Autodesk Fusion 360 part; units mm, degrees
note: some values were not read from the file. Set by a fixed rule: which sketch regions a step uses.
(part 2 of 2)
sketch "Sketch14" plane through (0, 1.4, 0) normal (0, 1, 0) x (-1, 0, 0)
  circle A0 centre (-36, -115) radius 1.625
  circle A1 centre (-3.5, -133) radius 1.625
  line L0 (0, -38.25) -> (-124, -38.25)
  line L1 (-124, -38.25) -> (-124, -58)
  line L2 (-124, -58) -> (-102, -112)
  line L3 (-102, -112) -> (-96.5, -117.5)
  line L4 (-96.5, -117.5) -> (-25, -136.5)
  line L5 (-25, -136.5) -> (-2.5, -136.5)
  line L6 (-2.5, -136.5) -> (0, -134)
  line L7 (0, -134) -> (0, -38.25)
  line L8 (-68.85, -56.1) -> (-82.85, -56.1)
  line L9 (-82.85, -56.1) -> (-82.85, -42.1)
  line L10 (-82.85, -42.1) -> (-68.85, -42.1)
  line L11 (-68.85, -42.1) -> (-68.85, -56.1)
  line L12 (-51, -56.1) -> (-65, -56.1)
  line L13 (-65, -56.1) -> (-65, -42.1)
  line L14 (-65, -42.1) -> (-51, -42.1)
  line L15 (-51, -42.1) -> (-51, -56.1)
  line L16 (-86.7, -56.1) -> (-100.7, -56.1)
  line L17 (-100.7, -56.1) -> (-100.7, -42.1)
  line L18 (-100.7, -42.1) -> (-86.7, -42.1)
  line L19 (-86.7, -42.1) -> (-86.7, -56.1)
  line L20 (-21.075, -56.1) -> (-35.075, -56.1)
  line L21 (-35.075, -56.1) -> (-35.075, -42.1)
  line L22 (-35.075, -42.1) -> (-21.075, -42.1)
  line L23 (-21.075, -42.1) -> (-21.075, -56.1)
  line L24 (-104.55, -56.1) -> (-118.55, -56.1)
  line L25 (-118.55, -56.1) -> (-118.55, -42.1)
  line L26 (-118.55, -42.1) -> (-104.55, -42.1)
  line L27 (-104.55, -42.1) -> (-104.55, -56.1)
  line L28 (-62.7, -73.95) -> (-76.7, -73.95)
  line L29 (-76.7, -73.95) -> (-76.7, -59.95)
  line L30 (-76.7, -59.95) -> (-62.7, -59.95)
  line L31 (-62.7, -59.95) -> (-62.7, -73.95)
  line L32 (-44.85, -59.95) -> (-44.85, -73.95)
  line L33 (-44.85, -73.95) -> (-58.85, -73.95)
  line L34 (-58.85, -73.95) -> (-58.85, -59.95)
  line L35 (-58.85, -59.95) -> (-44.85, -59.95)
  line L36 (-80.55, -73.95) -> (-94.55, -73.95)
  line L37 (-94.55, -73.95) -> (-94.55, -59.95)
  line L38 (-94.55, -59.95) -> (-80.55, -59.95)
  line L39 (-80.55, -59.95) -> (-80.55, -73.95)
  line L40 (-19.675, -73.95) -> (-33.675, -73.95)
  line L41 (-33.675, -73.95) -> (-33.675, -59.95)
  line L42 (-33.675, -59.95) -> (-19.675, -59.95)
  line L43 (-19.675, -59.95) -> (-19.675, -73.95)
  line L44 (-98.4, -59.95) -> (-98.4, -73.95)
  line L45 (-98.4, -73.95) -> (-112.4, -73.95)
  line L46 (-112.4, -73.95) -> (-112.4, -59.95)
  line L47 (-112.4, -59.95) -> (-98.4, -59.95)
  line L48 (-68.6, -91.85) -> (-68.6, -77.85)
  line L49 (-68.6, -77.85) -> (-54.6, -77.85)
  line L50 (-54.6, -77.85) -> (-54.6, -91.85)
  line L51 (-54.6, -91.85) -> (-68.6, -91.85)
  line L52 (-50.75, -91.85) -> (-50.75, -77.85)
  line L53 (-50.75, -77.85) -> (-36.75, -77.85)
  line L54 (-36.75, -77.85) -> (-36.75, -91.85)
  line L55 (-36.75, -91.85) -> (-50.75, -91.85)
  line L56 (-86.45, -91.85) -> (-86.45, -77.85)
  line L57 (-86.45, -77.85) -> (-72.45, -77.85)
  line L58 (-72.45, -77.85) -> (-72.45, -91.85)
  line L59 (-72.45, -91.85) -> (-86.45, -91.85)
  line L60 (-28.325, -77.85) -> (-14.325, -77.85)
  line L61 (-14.325, -77.85) -> (-14.325, -91.85)
  line L62 (-14.325, -91.85) -> (-28.325, -91.85)
  line L63 (-28.325, -91.85) -> (-28.325, -77.85)
  line L64 (-104.3, -91.85) -> (-104.3, -77.85)
  line L65 (-104.3, -77.85) -> (-90.3, -77.85)
  line L66 (-90.3, -77.85) -> (-90.3, -91.85)
  line L67 (-90.3, -91.85) -> (-104.3, -91.85)
  line L68 (-44.7, -95.65) -> (-44.7, -109.65)
  line L69 (-44.7, -109.65) -> (-58.7, -109.65)
  line L70 (-58.7, -109.65) -> (-58.7, -95.65)
  line L71 (-58.7, -95.65) -> (-44.7, -95.65)
  line L72 (-26.85, -95.65) -> (-26.85, -109.65)
  line L73 (-26.85, -109.65) -> (-40.85, -109.65)
  line L74 (-40.85, -109.65) -> (-40.85, -95.65)
  line L75 (-40.85, -95.65) -> (-26.85, -95.65)
  line L76 (-62.55, -95.65) -> (-62.55, -109.65)
  line L77 (-62.55, -109.65) -> (-76.55, -109.65)
  line L78 (-76.55, -109.65) -> (-76.55, -95.65)
  line L79 (-76.55, -95.65) -> (-62.55, -95.65)
  line L80 (-9, -95.65) -> (-9, -109.65)
  line L81 (-9, -109.65) -> (-23, -109.65)
  line L82 (-23, -109.65) -> (-23, -95.65)
  line L83 (-23, -95.65) -> (-9, -95.65)
  line L84 (-80.4, -95.65) -> (-80.4, -109.65)
  line L85 (-80.4, -109.65) -> (-94.4, -109.65)
  line L86 (-94.4, -109.65) -> (-94.4, -95.65)
  line L87 (-94.4, -95.65) -> (-80.4, -95.65)
  line L88 (-9, -113.5) -> (-9, -127.5)
  line L89 (-9, -127.5) -> (-23, -127.5)
  line L90 (-23, -127.5) -> (-23, -113.5)
  line L91 (-23, -113.5) -> (-9, -113.5)
  line L92 (0, -134) -> (0, -136.5)
  line L93 (0, -136.5) -> (-100, -136.5)
  line L94 (-100, -136.5) -> (-100, -97.5)
  line L95 (0, -136.5) -> (-110.5, -136.5)
  line L96 (-110.5, -136.5) -> (-110.5, -79.5)
  line L97 (0, -136.5) -> (-115, -136.5)
  line L98 (-115, -136.5) -> (-115, -62)
  circle A2 centre (-100, -97.5) radius 1.625
  circle A3 centre (-110.5, -79.5) radius 1.625
  circle A4 centre (-115, -62) radius 1.625
  line L99 (0, -67) -> (-23.5, -67)
  dimension "d114" = 100
  dimension "d115" = 39
  dimension "d116" = 110.5
  dimension "d117" = 57
  dimension "d118" = 74.5
  dimension "d119" = 3.25
  dimension "d120" = 3.25
  dimension "d121" = 3.25
  dimension "d122" = 23.5
  constraint coincident L6.end L7.start
  constraint perpendicular L5 L92
  constraint perpendicular L92 L93
  constraint perpendicular L93 L94
  constraint perpendicular L94 L95
  constraint perpendicular L95 L96
  constraint perpendicular L92 L97
  constraint perpendicular L97 L98
  constraint coincident L94.end A2.centre
  constraint coincident L96.end A3.centre
  constraint coincident L98.end A4.centre
  constraint coincident L7 L99.start
  constraint perpendicular L7 L99
  measures "d114" distance of L92.end L93.end
  measures "d115" distance of L93.end L94.end
  measures "d116" distance of L92.end L95.end
  measures "d117" distance of L95.end L96.end
  measures "d118" distance of L97.end L98.end
  measures "d119" diameter of A2
  measures "d120" diameter of A3
  measures "d121" diameter of A4
  measures "d122" distance of L99.start L99.end
extrude "Extrude14" cut sketch "Sketch14" against normal blind 5 contours A2 | A3 | A4
sketch "Sketch15" plane through (0, 1.4, 0) normal (0, 1, 0) x (-1, 0, 0)
  circle A0 centre (-100, -97.5) radius 1.625
  circle A1 centre (-110.5, -79.5) radius 1.625
  circle A2 centre (-115, -62) radius 1.625
  circle A3 centre (-36, -115) radius 1.625
  circle A4 centre (-3.5, -133) radius 1.625
  line L0 (0, -38.25) -> (-124, -38.25)
  line L1 (-124, -38.25) -> (-124, -58)
  line L2 (-124, -58) -> (-102, -112)
  line L3 (-102, -112) -> (-96.5, -117.5)
  line L4 (-96.5, -117.5) -> (-25, -136.5)
  line L5 (-25, -136.5) -> (-2.5, -136.5)
  line L6 (-2.5, -136.5) -> (0, -134)
  line L7 (0, -134) -> (0, -38.25)
  line L8 (-68.85, -56.1) -> (-82.85, -56.1)
  line L9 (-82.85, -56.1) -> (-82.85, -42.1)
  line L10 (-82.85, -42.1) -> (-68.85, -42.1)
  line L11 (-68.85, -42.1) -> (-68.85, -56.1)
  line L12 (-51, -56.1) -> (-65, -56.1)
  line L13 (-65, -56.1) -> (-65, -42.1)
  line L14 (-65, -42.1) -> (-51, -42.1)
  line L15 (-51, -42.1) -> (-51, -56.1)
  line L16 (-86.7, -56.1) -> (-100.7, -56.1)
  line L17 (-100.7, -56.1) -> (-100.7, -42.1)
  line L18 (-100.7, -42.1) -> (-86.7, -42.1)
  line L19 (-86.7, -42.1) -> (-86.7, -56.1)
  line L20 (-21.075, -56.1) -> (-35.075, -56.1)
  line L21 (-35.075, -56.1) -> (-35.075, -42.1)
  line L22 (-35.075, -42.1) -> (-21.075, -42.1)
  line L23 (-21.075, -42.1) -> (-21.075, -56.1)
  line L24 (-104.55, -56.1) -> (-118.55, -56.1)
  line L25 (-118.55, -56.1) -> (-118.55, -42.1)
  line L26 (-118.55, -42.1) -> (-104.55, -42.1)
  line L27 (-104.55, -42.1) -> (-104.55, -56.1)
  line L28 (-62.7, -73.95) -> (-76.7, -73.95)
  line L29 (-76.7, -73.95) -> (-76.7, -59.95)
  line L30 (-76.7, -59.95) -> (-62.7, -59.95)
  line L31 (-62.7, -59.95) -> (-62.7, -73.95)
  line L32 (-44.85, -59.95) -> (-44.85, -73.95)
  line L33 (-44.85, -73.95) -> (-58.85, -73.95)
  line L34 (-58.85, -73.95) -> (-58.85, -59.95)
  line L35 (-58.85, -59.95) -> (-44.85, -59.95)
  line L36 (-80.55, -73.95) -> (-94.55, -73.95)
  line L37 (-94.55, -73.95) -> (-94.55, -59.95)
  line L38 (-94.55, -59.95) -> (-80.55, -59.95)
  line L39 (-80.55, -59.95) -> (-80.55, -73.95)
  line L40 (-19.675, -73.95) -> (-33.675, -73.95)
  line L41 (-33.675, -73.95) -> (-33.675, -59.95)
  line L42 (-33.675, -59.95) -> (-19.675, -59.95)
  line L43 (-19.675, -59.95) -> (-19.675, -73.95)
  line L44 (-98.4, -59.95) -> (-98.4, -73.95)
  line L45 (-98.4, -73.95) -> (-112.4, -73.95)
  line L46 (-112.4, -73.95) -> (-112.4, -59.95)
  line L47 (-112.4, -59.95) -> (-98.4, -59.95)
  line L48 (-68.6, -91.85) -> (-68.6, -77.85)
  line L49 (-68.6, -77.85) -> (-54.6, -77.85)
  line L50 (-54.6, -77.85) -> (-54.6, -91.85)
  line L51 (-54.6, -91.85) -> (-68.6, -91.85)
  line L52 (-50.75, -91.85) -> (-50.75, -77.85)
  line L53 (-50.75, -77.85) -> (-36.75, -77.85)
  line L54 (-36.75, -77.85) -> (-36.75, -91.85)
  line L55 (-36.75, -91.85) -> (-50.75, -91.85)
  line L56 (-86.45, -91.85) -> (-86.45, -77.85)
  line L57 (-86.45, -77.85) -> (-72.45, -77.85)
  line L58 (-72.45, -77.85) -> (-72.45, -91.85)
  line L59 (-72.45, -91.85) -> (-86.45, -91.85)
  line L60 (-28.325, -77.85) -> (-14.325, -77.85)
  line L61 (-14.325, -77.85) -> (-14.325, -91.85)
  line L62 (-14.325, -91.85) -> (-28.325, -91.85)
  line L63 (-28.325, -91.85) -> (-28.325, -77.85)
  line L64 (-104.3, -91.85) -> (-104.3, -77.85)
  line L65 (-104.3, -77.85) -> (-90.3, -77.85)
  line L66 (-90.3, -77.85) -> (-90.3, -91.85)
  line L67 (-90.3, -91.85) -> (-104.3, -91.85)
  line L68 (-44.7, -95.65) -> (-44.7, -109.65)
  line L69 (-44.7, -109.65) -> (-58.7, -109.65)
  line L70 (-58.7, -109.65) -> (-58.7, -95.65)
  line L71 (-58.7, -95.65) -> (-44.7, -95.65)
  line L72 (-26.85, -95.65) -> (-26.85, -109.65)
  line L73 (-26.85, -109.65) -> (-40.85, -109.65)
  line L74 (-40.85, -109.65) -> (-40.85, -95.65)
  line L75 (-40.85, -95.65) -> (-26.85, -95.65)
  line L76 (-62.55, -95.65) -> (-62.55, -109.65)
  line L77 (-62.55, -109.65) -> (-76.55, -109.65)
  line L78 (-76.55, -109.65) -> (-76.55, -95.65)
  line L79 (-76.55, -95.65) -> (-62.55, -95.65)
  line L80 (-9, -95.65) -> (-9, -109.65)
  line L81 (-9, -109.65) -> (-23, -109.65)
  line L82 (-23, -109.65) -> (-23, -95.65)
  line L83 (-23, -95.65) -> (-9, -95.65)
  line L84 (-80.4, -95.65) -> (-80.4, -109.65)
  line L85 (-80.4, -109.65) -> (-94.4, -109.65)
  line L86 (-94.4, -109.65) -> (-94.4, -95.65)
  line L87 (-94.4, -95.65) -> (-80.4, -95.65)
  line L88 (-9, -113.5) -> (-9, -127.5)
  line L89 (-9, -127.5) -> (-23, -127.5)
  line L90 (-23, -127.5) -> (-23, -113.5)
  line L91 (-23, -113.5) -> (-9, -113.5)
extrude "Extrude15" add sketch "Sketch15" against normal blind 1.4 contours L28 L29 L30 L31 | L32 L33 L34 L35 | L36 L37 L38 L39 | L40 L41 L42 L43 | L44 L45 L46 L47
sketch "Sketch16" plane through (0, 1.4, 0) normal (0, 1, 0) x (-1, 0, 0)
  circle A0 centre (-100, -97.5) radius 1.625
  circle A1 centre (-110.5, -79.5) radius 1.625
  circle A2 centre (-115, -62) radius 1.625
  circle A3 centre (-36, -115) radius 1.625
  circle A4 centre (-3.5, -133) radius 1.625
  line L0 (0, -38.25) -> (-124, -38.25)
  line L1 (-124, -38.25) -> (-124, -58)
  line L2 (-124, -58) -> (-102, -112)
  line L3 (-102, -112) -> (-96.5, -117.5)
  line L4 (-96.5, -117.5) -> (-25, -136.5)
  line L5 (-25, -136.5) -> (-2.5, -136.5)
  line L6 (-2.5, -136.5) -> (0, -134)
  line L7 (0, -134) -> (0, -38.25)
  line L8 (-68.85, -56.1) -> (-82.85, -56.1)
  line L9 (-82.85, -56.1) -> (-82.85, -42.1)
  line L10 (-82.85, -42.1) -> (-68.85, -42.1)
  line L11 (-68.85, -42.1) -> (-68.85, -56.1)
  line L12 (-51, -56.1) -> (-65, -56.1)
  line L13 (-65, -56.1) -> (-65, -42.1)
  line L14 (-65, -42.1) -> (-51, -42.1)
  line L15 (-51, -42.1) -> (-51, -56.1)
  line L16 (-86.7, -56.1) -> (-100.7, -56.1)
  line L17 (-100.7, -56.1) -> (-100.7, -42.1)
  line L18 (-100.7, -42.1) -> (-86.7, -42.1)
  line L19 (-86.7, -42.1) -> (-86.7, -56.1)
  line L20 (-21.075, -56.1) -> (-35.075, -56.1)
  line L21 (-35.075, -56.1) -> (-35.075, -42.1)
  line L22 (-35.075, -42.1) -> (-21.075, -42.1)
  line L23 (-21.075, -42.1) -> (-21.075, -56.1)
  line L24 (-104.55, -56.1) -> (-118.55, -56.1)
  line L25 (-118.55, -56.1) -> (-118.55, -42.1)
  line L26 (-118.55, -42.1) -> (-104.55, -42.1)
  line L27 (-104.55, -42.1) -> (-104.55, -56.1)
  line L28 (-68.6, -91.85) -> (-68.6, -77.85)
  line L29 (-68.6, -77.85) -> (-54.6, -77.85)
  line L30 (-54.6, -77.85) -> (-54.6, -91.85)
  line L31 (-54.6, -91.85) -> (-68.6, -91.85)
  line L32 (-50.75, -91.85) -> (-50.75, -77.85)
  line L33 (-50.75, -77.85) -> (-36.75, -77.85)
  line L34 (-36.75, -77.85) -> (-36.75, -91.85)
  line L35 (-36.75, -91.85) -> (-50.75, -91.85)
  line L36 (-86.45, -91.85) -> (-86.45, -77.85)
  line L37 (-86.45, -77.85) -> (-72.45, -77.85)
  line L38 (-72.45, -77.85) -> (-72.45, -91.85)
  line L39 (-72.45, -91.85) -> (-86.45, -91.85)
  line L40 (-28.325, -77.85) -> (-14.325, -77.85)
  line L41 (-14.325, -77.85) -> (-14.325, -91.85)
  line L42 (-14.325, -91.85) -> (-28.325, -91.85)
  line L43 (-28.325, -91.85) -> (-28.325, -77.85)
  line L44 (-104.3, -91.85) -> (-104.3, -77.85)
  line L45 (-104.3, -77.85) -> (-90.3, -77.85)
  line L46 (-90.3, -77.85) -> (-90.3, -91.85)
  line L47 (-90.3, -91.85) -> (-104.3, -91.85)
  line L48 (-44.7, -95.65) -> (-44.7, -109.65)
  line L49 (-44.7, -109.65) -> (-58.7, -109.65)
  line L50 (-58.7, -109.65) -> (-58.7, -95.65)
  line L51 (-58.7, -95.65) -> (-44.7, -95.65)
  line L52 (-26.85, -95.65) -> (-26.85, -109.65)
  line L53 (-26.85, -109.65) -> (-40.85, -109.65)
  line L54 (-40.85, -109.65) -> (-40.85, -95.65)
  line L55 (-40.85, -95.65) -> (-26.85, -95.65)
  line L56 (-62.55, -95.65) -> (-62.55, -109.65)
  line L57 (-62.55, -109.65) -> (-76.55, -109.65)
  line L58 (-76.55, -109.65) -> (-76.55, -95.65)
  line L59 (-76.55, -95.65) -> (-62.55, -95.65)
  line L60 (-9, -95.65) -> (-9, -109.65)
  line L61 (-9, -109.65) -> (-23, -109.65)
  line L62 (-23, -109.65) -> (-23, -95.65)
  line L63 (-23, -95.65) -> (-9, -95.65)
  line L64 (-80.4, -95.65) -> (-80.4, -109.65)
  line L65 (-80.4, -109.65) -> (-94.4, -109.65)
  line L66 (-94.4, -109.65) -> (-94.4, -95.65)
  line L67 (-94.4, -95.65) -> (-80.4, -95.65)
  line L68 (-9, -113.5) -> (-9, -127.5)
  line L69 (-9, -127.5) -> (-23, -127.5)
  line L70 (-23, -127.5) -> (-23, -113.5)
  line L71 (-23, -113.5) -> (-9, -113.5)
  line L72 (0, -66.975) -> (-23.5, -66.975)
  line L73 (-30.5, -73.975) -> (-16.5, -73.975)
  line L74 (-16.5, -73.975) -> (-16.5, -59.975)
  line L75 (-16.5, -59.975) -> (-30.5, -59.975)
  line L76 (-30.5, -59.975) -> (-30.5, -73.975)
  line L77 (-30.5, -73.975) -> (-16.5, -59.975) construction
  line L78 (-16.5, -73.975) -> (-30.5, -59.975) construction
  line L79 (-23.5, -66.975) -> (-48.675, -66.975)
  line L80 (-55.675, -73.975) -> (-41.675, -73.975)
  line L81 (-41.675, -73.975) -> (-41.675, -59.975)
  line L82 (-41.675, -59.975) -> (-55.675, -59.975)
  line L83 (-55.675, -59.975) -> (-55.675, -73.975)
  line L84 (-55.675, -73.975) -> (-41.675, -59.975) construction
  line L85 (-41.675, -73.975) -> (-55.675, -59.975) construction
  line L86 (-48.675, -66.975) -> (-66.525, -66.975)
  line L87 (-66.525, -66.975) -> (-84.375, -66.975)
  line L88 (-84.375, -66.975) -> (-102.225, -66.975)
  line L89 (-59.525, -59.975) -> (-73.525, -59.975)
  line L90 (-73.525, -59.975) -> (-73.525, -73.975)
  line L91 (-73.525, -73.975) -> (-59.525, -73.975)
  line L92 (-59.525, -73.975) -> (-59.525, -59.975)
  line L93 (-59.525, -59.975) -> (-73.525, -73.975) construction
  line L94 (-73.525, -59.975) -> (-59.525, -73.975) construction
  line L95 (-91.375, -73.975) -> (-77.375, -73.975)
  line L96 (-77.375, -73.975) -> (-77.375, -59.975)
  line L97 (-77.375, -59.975) -> (-91.375, -59.975)
  line L98 (-91.375, -59.975) -> (-91.375, -73.975)
  line L99 (-91.375, -73.975) -> (-77.375, -59.975) construction
  line L100 (-77.375, -73.975) -> (-91.375, -59.975) construction
  line L101 (-109.225, -73.975) -> (-95.225, -73.975)
  line L102 (-95.225, -73.975) -> (-95.225, -59.975)
  line L103 (-95.225, -59.975) -> (-109.225, -59.975)
  line L104 (-109.225, -59.975) -> (-109.225, -73.975)
  line L105 (-109.225, -73.975) -> (-95.225, -59.975) construction
  line L106 (-95.225, -73.975) -> (-109.225, -59.975) construction
  point P0 (-23.5, -66.975)
  point P1 (-48.675, -66.975)
  point P2 (-66.525, -66.975)
  point P3 (-84.375, -66.975)
  point P4 (-102.225, -66.975)
  dimension "d127" = 23.5
  dimension "d128" = 14
  dimension "d129" = 14
  dimension "d130" = 25.175
  dimension "d131" = 14
  dimension "d132" = 14
  dimension "d133" = 17.85
  dimension "d134" = 17.85
  dimension "d135" = 17.85
  dimension "d136" = 14
  dimension "d137" = 14
  dimension "d138" = 14
  dimension "d139" = 14
  dimension "d140" = 14
  dimension "d141" = 14
  constraint perpendicular L7 L72
  constraint horizontal L73
  constraint perpendicular L73 L74
  constraint parallel L73 L75
  constraint parallel L74 L76
  constraint coincident L77 P0
  constraint coincident L78 P0
  constraint coincident P0 L72.end
  constraint perpendicular L76 L79
  constraint horizontal L80
  constraint perpendicular L80 L81
  constraint parallel L80 L82
  constraint parallel L81 L83
  constraint coincident L84 P1
  constraint coincident L85 P1
  constraint coincident P1 L79.end
  constraint perpendicular L83 L86
  constraint parallel L86 L87
  constraint parallel L87 L88
  constraint horizontal L89
  constraint perpendicular L89 L90
  constraint parallel L89 L91
  constraint parallel L90 L92
  constraint coincident L93 P2
  constraint coincident L94 P2
  constraint coincident P2 L86.end
  constraint horizontal L95
  constraint perpendicular L95 L96
  constraint parallel L95 L97
  constraint parallel L96 L98
  constraint coincident L99 P3
  constraint coincident L100 P3
  constraint coincident P3 L87.end
  constraint horizontal L101
  constraint perpendicular L101 L102
  constraint parallel L101 L103
  constraint parallel L102 L104
  constraint coincident L105 P4
  constraint coincident L106 P4
  constraint coincident P4 L88.end
  measures "d127" distance of L72.start P0
  measures "d128" distance of L74.end L75.end
  measures "d129" distance of L73.end L74.end
  measures "d130" distance of P0 P1
  measures "d131" distance of L81.end L82.end
  measures "d132" distance of L80.end L81.end
  measures "d133" distance of P1 P2
  measures "d134" distance of P2 P3
  measures "d135" distance of P3 P4
  measures "d136" distance of L90.end L91.end
  measures "d137" distance of L89.end L90.end
  measures "d138" distance of L96.end L97.end
  measures "d139" distance of L95.end L96.end
  measures "d140" distance of L102.end L103.end
  measures "d141" distance of L101.end L102.end
extrude "Extrude16" cut sketch "Sketch16" against normal blind 5 contours L72 L73 L74 L76 L79 | L72 L74 L75 L76 L79 | L79 L80 L81 L83 L86 | L79 L81 L82 L83 L86 | L86 L87 L90 L91 L92 | L86 L87 L89 L90 L92 | L87 L88 L95 L96 L98 | L87 L88 L96 L97 L98 | L101 L102 L103 L104
sketch "Sketch17" plane through (0, 1.4, 0) normal (0, 1, 0) x (-1, 0, 0)
  line L0 (-73.525, -59.975) -> (-59.525, -59.975)
  line L1 (-59.525, -59.975) -> (-59.525, -73.975)
  line L2 (-59.525, -73.975) -> (-73.525, -73.975)
  line L3 (-73.525, -73.975) -> (-73.525, -59.975)
  line L4 (-77.375, -73.975) -> (-91.375, -73.975)
  line L5 (-91.375, -73.975) -> (-91.375, -59.975)
  line L6 (-91.375, -59.975) -> (-77.375, -59.975)
  line L7 (-77.375, -59.975) -> (-77.375, -73.975)
  line L8 (-41.675, -73.975) -> (-55.675, -73.975)
  line L9 (-55.675, -73.975) -> (-55.675, -59.975)
  line L10 (-55.675, -59.975) -> (-41.675, -59.975)
  line L11 (-41.675, -59.975) -> (-41.675, -73.975)
  line L12 (-95.225, -73.975) -> (-109.225, -73.975)
  line L13 (-109.225, -73.975) -> (-109.225, -59.975)
  line L14 (-109.225, -59.975) -> (-95.225, -59.975)
  line L15 (-95.225, -59.975) -> (-95.225, -73.975)
  line L16 (-16.5, -73.975) -> (-30.5, -73.975)
  line L17 (-30.5, -73.975) -> (-30.5, -59.975)
  line L18 (-30.5, -59.975) -> (-16.5, -59.975)
  line L19 (-16.5, -59.975) -> (-16.5, -73.975)
  circle A0 centre (-100, -97.5) radius 1.625
  circle A1 centre (-110.5, -79.5) radius 1.625
  circle A2 centre (-115, -62) radius 1.625
  circle A3 centre (-36, -115) radius 1.625
  circle A4 centre (-3.5, -133) radius 1.625
  line L20 (0, -38.25) -> (-124, -38.25)
  line L21 (-124, -38.25) -> (-124, -58)
  line L22 (-124, -58) -> (-102, -112)
  line L23 (-102, -112) -> (-96.5, -117.5)
  line L24 (-96.5, -117.5) -> (-25, -136.5)
  line L25 (-25, -136.5) -> (-2.5, -136.5)
  line L26 (-2.5, -136.5) -> (0, -134)
  line L27 (0, -134) -> (0, -38.25)
  line L28 (-68.85, -56.1) -> (-82.85, -56.1)
  line L29 (-82.85, -56.1) -> (-82.85, -42.1)
  line L30 (-82.85, -42.1) -> (-68.85, -42.1)
  line L31 (-68.85, -42.1) -> (-68.85, -56.1)
  line L32 (-51, -56.1) -> (-65, -56.1)
  line L33 (-65, -56.1) -> (-65, -42.1)
  line L34 (-65, -42.1) -> (-51, -42.1)
  line L35 (-51, -42.1) -> (-51, -56.1)
  line L36 (-86.7, -56.1) -> (-100.7, -56.1)
  line L37 (-100.7, -56.1) -> (-100.7, -42.1)
  line L38 (-100.7, -42.1) -> (-86.7, -42.1)
  line L39 (-86.7, -42.1) -> (-86.7, -56.1)
  line L40 (-21.075, -56.1) -> (-35.075, -56.1)
  line L41 (-35.075, -56.1) -> (-35.075, -42.1)
  line L42 (-35.075, -42.1) -> (-21.075, -42.1)
  line L43 (-21.075, -42.1) -> (-21.075, -56.1)
  line L44 (-104.55, -56.1) -> (-118.55, -56.1)
  line L45 (-118.55, -56.1) -> (-118.55, -42.1)
  line L46 (-118.55, -42.1) -> (-104.55, -42.1)
  line L47 (-104.55, -42.1) -> (-104.55, -56.1)
  line L48 (-68.6, -91.85) -> (-68.6, -77.85)
  line L49 (-68.6, -77.85) -> (-54.6, -77.85)
  line L50 (-54.6, -77.85) -> (-54.6, -91.85)
  line L51 (-54.6, -91.85) -> (-68.6, -91.85)
  line L52 (-50.75, -91.85) -> (-50.75, -77.85)
  line L53 (-50.75, -77.85) -> (-36.75, -77.85)
  line L54 (-36.75, -77.85) -> (-36.75, -91.85)
  line L55 (-36.75, -91.85) -> (-50.75, -91.85)
  line L56 (-86.45, -91.85) -> (-86.45, -77.85)
  line L57 (-86.45, -77.85) -> (-72.45, -77.85)
  line L58 (-72.45, -77.85) -> (-72.45, -91.85)
  line L59 (-72.45, -91.85) -> (-86.45, -91.85)
  line L60 (-28.325, -77.85) -> (-14.325, -77.85)
  line L61 (-14.325, -77.85) -> (-14.325, -91.85)
  line L62 (-14.325, -91.85) -> (-28.325, -91.85)
  line L63 (-28.325, -91.85) -> (-28.325, -77.85)
  line L64 (-104.3, -91.85) -> (-104.3, -77.85)
  line L65 (-104.3, -77.85) -> (-90.3, -77.85)
  line L66 (-90.3, -77.85) -> (-90.3, -91.85)
  line L67 (-90.3, -91.85) -> (-104.3, -91.85)
  line L68 (-44.7, -95.65) -> (-44.7, -109.65)
  line L69 (-44.7, -109.65) -> (-58.7, -109.65)
  line L70 (-58.7, -109.65) -> (-58.7, -95.65)
  line L71 (-58.7, -95.65) -> (-44.7, -95.65)
  line L72 (-26.85, -95.65) -> (-26.85, -109.65)
  line L73 (-26.85, -109.65) -> (-40.85, -109.65)
  line L74 (-40.85, -109.65) -> (-40.85, -95.65)
  line L75 (-40.85, -95.65) -> (-26.85, -95.65)
  line L76 (-62.55, -95.65) -> (-62.55, -109.65)
  line L77 (-62.55, -109.65) -> (-76.55, -109.65)
  line L78 (-76.55, -109.65) -> (-76.55, -95.65)
  line L79 (-76.55, -95.65) -> (-62.55, -95.65)
  line L80 (-9, -95.65) -> (-9, -109.65)
  line L81 (-9, -109.65) -> (-23, -109.65)
  line L82 (-23, -109.65) -> (-23, -95.65)
  line L83 (-23, -95.65) -> (-9, -95.65)
  line L84 (-80.4, -95.65) -> (-80.4, -109.65)
  line L85 (-80.4, -109.65) -> (-94.4, -109.65)
  line L86 (-94.4, -109.65) -> (-94.4, -95.65)
  line L87 (-94.4, -95.65) -> (-80.4, -95.65)
  line L88 (-9, -113.5) -> (-9, -127.5)
  line L89 (-9, -127.5) -> (-23, -127.5)
  line L90 (-23, -127.5) -> (-23, -113.5)
  line L91 (-23, -113.5) -> (-9, -113.5)
  line L92 (0, -38.25) -> (0, -40.75)
  line L93 (0, -38.25) -> (-2.5, -38.25)
  line L94 (-2.5, -38.25) -> (0, -40.75)
  line L95 (-124, -38.25) -> (-121.5, -38.25)
  line L96 (-124, -38.25) -> (-124, -40.75)
  line L97 (-124, -40.75) -> (-121.5, -38.25)
  dimension "d144" = 2.5
  dimension "d145" = 2.5
  dimension "d146" = 2.5
  dimension "d147" = 2.5
  constraint coincident L20.start L27.end
  constraint perpendicular L20 L92
  constraint perpendicular L27 L93
  constraint coincident L20.end L21.start
  constraint perpendicular L27 L95
  constraint perpendicular L95 L96
  measures "d144" distance of L20.start L92.end
  measures "d145" distance of L20.start L93.end
  measures "d146" distance of L20.end L95.end
  measures "d147" distance of L20.end L96.end
extrude "Extrude17" cut sketch "Sketch17" against normal blind 5 contours L20 L27 L92 L93 L94 | L20 L21 L95 L96 L97
sketch "Sketch18" plane through (0, 1.4, 0) normal (0, 1, 0) x (-1, 0, 0)
  line L0 (-121.5, -38.25) -> (-124, -40.75)
  line L1 (-124, -40.75) -> (-124, -58)
  line L2 (-124, -58) -> (-102, -112)
  line L3 (-102, -112) -> (-96.5, -117.5)
  line L4 (-96.5, -117.5) -> (-25, -136.5)
  line L5 (-25, -136.5) -> (-2.5, -136.5)
  line L6 (-2.5, -136.5) -> (0, -134)
  line L7 (0, -134) -> (0, -40.75)
  line L8 (0, -40.75) -> (-2.5, -38.25)
  line L9 (-2.5, -38.25) -> (-121.5, -38.25)
  line L10 (-73.525, -59.975) -> (-59.525, -59.975)
  line L11 (-59.525, -59.975) -> (-59.525, -73.975)
  line L12 (-59.525, -73.975) -> (-73.525, -73.975)
  line L13 (-73.525, -73.975) -> (-73.525, -59.975)
  line L14 (-77.375, -73.975) -> (-91.375, -73.975)
  line L15 (-91.375, -73.975) -> (-91.375, -59.975)
  line L16 (-91.375, -59.975) -> (-77.375, -59.975)
  line L17 (-77.375, -59.975) -> (-77.375, -73.975)
  line L18 (-41.675, -73.975) -> (-55.675, -73.975)
  line L19 (-55.675, -73.975) -> (-55.675, -59.975)
  line L20 (-55.675, -59.975) -> (-41.675, -59.975)
  line L21 (-41.675, -59.975) -> (-41.675, -73.975)
  line L22 (-95.225, -73.975) -> (-109.225, -73.975)
  line L23 (-109.225, -73.975) -> (-109.225, -59.975)
  line L24 (-109.225, -59.975) -> (-95.225, -59.975)
  line L25 (-95.225, -59.975) -> (-95.225, -73.975)
  line L26 (-16.5, -73.975) -> (-30.5, -73.975)
  line L27 (-30.5, -73.975) -> (-30.5, -59.975)
  line L28 (-30.5, -59.975) -> (-16.5, -59.975)
  line L29 (-16.5, -59.975) -> (-16.5, -73.975)
  circle A0 centre (-100, -97.5) radius 1.625
  circle A1 centre (-110.5, -79.5) radius 1.625
  circle A2 centre (-115, -62) radius 1.625
  circle A3 centre (-36, -115) radius 1.625
  circle A4 centre (-3.5, -133) radius 1.625
  line L30 (-68.85, -56.1) -> (-82.85, -56.1)
  line L31 (-82.85, -56.1) -> (-82.85, -42.1)
  line L32 (-82.85, -42.1) -> (-68.85, -42.1)
  line L33 (-68.85, -42.1) -> (-68.85, -56.1)
  line L34 (-51, -56.1) -> (-65, -56.1)
  line L35 (-65, -56.1) -> (-65, -42.1)
  line L36 (-65, -42.1) -> (-51, -42.1)
  line L37 (-51, -42.1) -> (-51, -56.1)
  line L38 (-86.7, -56.1) -> (-100.7, -56.1)
  line L39 (-100.7, -56.1) -> (-100.7, -42.1)
  line L40 (-100.7, -42.1) -> (-86.7, -42.1)
  line L41 (-86.7, -42.1) -> (-86.7, -56.1)
  line L42 (-21.075, -56.1) -> (-35.075, -56.1)
  line L43 (-35.075, -56.1) -> (-35.075, -42.1)
  line L44 (-35.075, -42.1) -> (-21.075, -42.1)
  line L45 (-21.075, -42.1) -> (-21.075, -56.1)
  line L46 (-104.55, -56.1) -> (-118.55, -56.1)
  line L47 (-118.55, -56.1) -> (-118.55, -42.1)
  line L48 (-118.55, -42.1) -> (-104.55, -42.1)
  line L49 (-104.55, -42.1) -> (-104.55, -56.1)
  line L50 (-68.6, -91.85) -> (-68.6, -77.85)
  line L51 (-68.6, -77.85) -> (-54.6, -77.85)
  line L52 (-54.6, -77.85) -> (-54.6, -91.85)
  line L53 (-54.6, -91.85) -> (-68.6, -91.85)
  line L54 (-50.75, -91.85) -> (-50.75, -77.85)
  line L55 (-50.75, -77.85) -> (-36.75, -77.85)
  line L56 (-36.75, -77.85) -> (-36.75, -91.85)
  line L57 (-36.75, -91.85) -> (-50.75, -91.85)
  line L58 (-86.45, -91.85) -> (-86.45, -77.85)
  line L59 (-86.45, -77.85) -> (-72.45, -77.85)
  line L60 (-72.45, -77.85) -> (-72.45, -91.85)
  line L61 (-72.45, -91.85) -> (-86.45, -91.85)
  line L62 (-28.325, -77.85) -> (-14.325, -77.85)
  line L63 (-14.325, -77.85) -> (-14.325, -91.85)
  line L64 (-14.325, -91.85) -> (-28.325, -91.85)
  line L65 (-28.325, -91.85) -> (-28.325, -77.85)
  line L66 (-104.3, -91.85) -> (-104.3, -77.85)
  line L67 (-104.3, -77.85) -> (-90.3, -77.85)
  line L68 (-90.3, -77.85) -> (-90.3, -91.85)
  line L69 (-90.3, -91.85) -> (-104.3, -91.85)
  line L70 (-44.7, -95.65) -> (-44.7, -109.65)
  line L71 (-44.7, -109.65) -> (-58.7, -109.65)
  line L72 (-58.7, -109.65) -> (-58.7, -95.65)
  line L73 (-58.7, -95.65) -> (-44.7, -95.65)
  line L74 (-26.85, -95.65) -> (-26.85, -109.65)
  line L75 (-26.85, -109.65) -> (-40.85, -109.65)
  line L76 (-40.85, -109.65) -> (-40.85, -95.65)
  line L77 (-40.85, -95.65) -> (-26.85, -95.65)
  line L78 (-62.55, -95.65) -> (-62.55, -109.65)
  line L79 (-62.55, -109.65) -> (-76.55, -109.65)
  line L80 (-76.55, -109.65) -> (-76.55, -95.65)
  line L81 (-76.55, -95.65) -> (-62.55, -95.65)
  line L82 (-9, -95.65) -> (-9, -109.65)
  line L83 (-9, -109.65) -> (-23, -109.65)
  line L84 (-23, -109.65) -> (-23, -95.65)
  line L85 (-23, -95.65) -> (-9, -95.65)
  line L86 (-80.4, -95.65) -> (-80.4, -109.65)
  line L87 (-80.4, -109.65) -> (-94.4, -109.65)
  line L88 (-94.4, -109.65) -> (-94.4, -95.65)
  line L89 (-94.4, -95.65) -> (-80.4, -95.65)
  line L90 (-9, -113.5) -> (-9, -127.5)
  line L91 (-9, -127.5) -> (-23, -127.5)
  line L92 (-23, -127.5) -> (-23, -113.5)
  line L93 (-23, -113.5) -> (-9, -113.5)
  line L94 (0, -38.25) -> (-3.5, -38.25)
  line L95 (-3.5, -38.25) -> (-3.5, -41.75)
  circle A5 centre (-3.5, -41.75) radius 1.625
  dimension "d150" = 3.5
  dimension "d151" = 3.5
  dimension "d152" = 3.25
  constraint parallel L9 L94
  constraint perpendicular L9 L95
  constraint coincident L95.end A5.centre
  measures "d150" distance of L94.start L94.end
  measures "d151" distance of L94.end L95.end
  measures "d152" diameter of A5
extrude "Extrude18" cut sketch "Sketch18" against normal blind 5 contours A5
equation "d53 = ( 27 / 2 ) * 1 mm + ( 17.85 / 2 ) * 1 mm"
equation "d67 = ( 17.85 / 0.5 ) * 1 mm"
equation "d68 = ( 32.5 / 2 ) * 1 mm - ( 17.85 / 2 ) * 1 mm"
equation "d71 = ( 32.5 / 2 ) * 1 mm + ( 17.85 / 2 ) * 1 mm"
equation "d85 = ( 17.85 / 0.25 ) * 1 mm"
equation "d86 = ( 42 / 2 ) * 1 mm - ( 17.85 / 2 ) * 1 mm"
equation "d89 = 21 mm + ( 17.85 / 2 ) * 1 mm"
equation "d130 = ( 32.5 / 2 ) * 1 mm + ( 17.85 / 2 ) * 1 mm"
